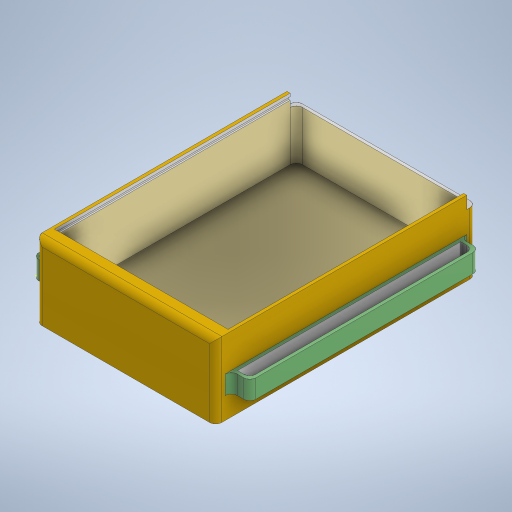
# Autodesk Inventor part: top
Saved by Autodesk Inventor 2023 (Build 270158000, 158)
## iProperties
Created: 2023-01-13
Part Number: top
Material: Generic
Document SubType Name: Modeling
Designer: zhanj390
Density: 1 g/cm^3
Appearance: Default
Author: zhanj390
Autodesk Inventor part; units mm, degrees
sketch "Sketch2" plane through (0, 0, 0) normal (0, 1, 0) x (-1, 0, 0)
  line L0 (0, 0) -> (-58, 0)
  line L1 (-58, 0) -> (-58, -84)
  line L2 (-58, -84) -> (0, -84)
  line L3 (0, -84) -> (0, 0)
  dimension "d0" = 58
  dimension "d1" = 84
  constraints: 8 end point, 2 parallel, 1 horizontal, 1 perpendicular
  measures "d0" distance of L1.end L2.end
  measures "d1" distance of L0.end L1.end
extrude "Extrusion1" add sketch "Sketch2" along normal blind 20
sketch "Sketch3" plane through (0, 20, 0) normal (0, 1, 0) x (1, 0, 0)
  line L0 (1, 1) -> (57, 1)
  line L1 (57, 1) -> (57, 83)
  line L2 (57, 83) -> (1, 83)
  line L3 (1, 83) -> (1, 1)
  line L4 (0, 84) -> (0, 0) projected
  line L5 (0, 0) -> (58, 0) projected
  line L6 (58, 84) -> (0, 84) projected
  line L7 (58, 0) -> (58, 84) projected
  dimension "d4" = 1
  dimension "d5" = 1
  dimension "d6" = 1
  dimension "d7" = 1
  constraints: 8 end point, 2 parallel, 1 horizontal, 1 perpendicular
  measures "d4" distance between parallel lines of L4 L3
  measures "d5" distance between parallel lines of L5 L0
  measures "d6" distance between parallel lines of L6 L2
  measures "d7" distance between parallel lines of L7 L1
extrude "Extrusion2" cut sketch "Sketch3" against normal blind 16 contours L3 L2 L1 L0
fillet "Fillet1" radius 2 4 edges at (0, 10, 0) (58, 10, 0) (58, 10, -84) (0, 10, -84)
ref_plane "Work Plane1" through (28, 20, -83) normal (-1, 0, 0) x (0, 0, 1)
sketch "Sketch17" plane through (58, 0, -2) normal (1, 0, 0) x (0, 0, -1)
  line L0 (3, 13) -> (77, 13)
  line L1 (77, 13) -> (77, 7)
  line L2 (77, 7) -> (3, 7)
  line L3 (3, 7) -> (3, 13)
  line L4 (0, 20) -> (80, 20) projected
  line L5 (0, 0) -> (80, 0) projected
  line L6 (80, 20) -> (80, 0) projected
  line L7 (0, 0) -> (0, 20) projected
  point P0 (-2, 0)
  point P1 (80, 10)
  point P2 (77, 10)
  point P3 (3, 10)
  dimension "d66" = 7
  dimension "d67" = 7
  dimension "d68" = 3
  dimension "d69" = 3
  constraints: 8 end point, 3 midpoint, 2 parallel, 1 horizontal, 1 perpendicular
  measures "d66" distance between parallel lines of L4 L0
  measures "d67" distance between parallel lines of L5 L2
  measures "d68" distance of point (80, 10) point (77, 10)
  measures "d69" distance from line of L7 point (3, 10)
extrude "Extrusion8" add sketch "Sketch17" along normal blind 6 contours L0 L1 L2 L3
sketch "Sketch18" plane through (58, 13, -5) normal (0, 1, 0) x (1, 0, 0)
  point P0 (-58, -5)
sketch "Sketch19" plane through (58, 13, -5) normal (0, 1, 0) x (1, 0, 0)
  line L0 (1, 73) -> (5, 73)
  line L1 (5, 73) -> (5, 1)
  line L2 (5, 1) -> (1, 1)
  line L3 (1, 1) -> (1, 73)
  line L4 (6, 74) -> (6, 0) projected
  line L5 (0, 0) -> (0, 74) projected
  line L6 (0, 0) -> (6, 0) projected
  line L7 (0, 74) -> (6, 74) projected
  point P0 (-58, -5)
  point P1 (3, 1)
  point P2 (3, 74)
  point P3 (3, 73)
  dimension "d72" = 1
  dimension "d73" = 1
  dimension "d74" = 1
  dimension "d75" = 1
  constraints: 8 end point, 3 midpoint, 2 parallel, 1 horizontal, 1 perpendicular
  measures "d72" distance between parallel lines of L4 L1
  measures "d73" distance between parallel lines of L5 L3
  measures "d74" distance from line of L6 point (3, 1)
  measures "d75" distance of point (3, 74) point (3, 73)
extrude "Extrusion9" cut sketch "Sketch19" against normal blind 6 contours L0 L1 L2 L3
fillet "Fillet4" radius 2 6 edges at (64, 10, -5) (64, 10, -79) (58, 10, -5) (58, 10, -79) (63, 10, -78) (63, 10, -6)
fillet "Fillet5" radius 2 4 edges at (1, 12, -83) (57, 12, -83) (57, 12, -1) (1, 12, -1)
ref_plane "Work Plane4" through (29, 0, -82) normal (-1, 0, 0) x (0, 0, 1)
mirror "Mirror2" about plane through (29, 0, -82) normal (-1, 0, 0) of "Extrusion8"
sketch "Sketch20" plane through (-6, 13, -79) normal (0, 1, 0) x (1, 0, 0)
  line L0 (5, -73) -> (1, -73)
  line L1 (1, -73) -> (1, -1)
  line L2 (1, -1) -> (5, -1)
  line L3 (5, -1) -> (5, -73)
  line L4 (6, -74) -> (0, -74) projected
  line L5 (0, 0) -> (0, -74) projected
  line L6 (6, 0) -> (6, -74) projected
  line L7 (6, 0) -> (0, 0) projected
  point P0 (6, -79)
  point P1 (3, -73)
  point P2 (3, -1)
  dimension "d80" = 1
  dimension "d81" = 1
  dimension "d82" = 1
  dimension "d83" = 1
  constraints: 8 end point, 2 midpoint, 2 parallel, 1 horizontal, 1 perpendicular
  measures "d80" distance from line of L4 point (3, -73)
  measures "d81" distance between parallel lines of L5 L1
  measures "d82" distance between parallel lines of L6 L3
  measures "d83" distance from line of L7 point (3, -1)
extrude "Extrusion10" cut sketch "Sketch20" against normal blind 6 contours L0 L1 L2 L3
fillet "Fillet6" radius 2 2 edges at (-6, 10, -5) (0, 10, -5)
fillet "Fillet7" radius 2 2 edges at (-6, 10, -79) (0, 10, -79)
ref_plane "Work Plane5" through (0, 20, 0) normal (0, 1, 0) x (1, 0, 0)
sketch "Sketch21" plane through (0, 20, 0) normal (0, 1, 0) x (1, 0, 0)
  line L0 (0, 82) -> (0, 2) projected
  line L1 (58, 0) -> (0, 0)
  line L2 (0, 0) -> (0, 5)
  line L3 (0, 5) -> (58, 5)
  line L4 (58, 5) -> (58, 0)
  line L5 (55, 1) -> (3, 1) projected
  line L6 (57, 81) -> (57, 3) projected
  line L7 (58, 5) -> (57, 5)
  line L8 (57, 5) -> (57, 81)
  line L9 (57, 81) -> (58, 81)
  line L10 (58, 81) -> (58, 5)
  line L11 (1, 3) -> (1, 81) projected
  line L12 (0, 5) -> (1, 5)
  line L13 (1, 5) -> (1, 81)
  line L14 (1, 81) -> (0, 81)
  line L15 (0, 81) -> (0, 5)
  point P0 (0, 0)
  point P1 (58, 2.5)
  point P2 (57, 5)
  point P3 (1, 5)
  point P4 (0, 81)
  dimension "d89" = 5
  dimension "d90" = 58
  dimension "d91" = 1
  constraints: 24 end point, 6 parallel, 3 horizontal, 3 perpendicular, 1 midpoint, 1 point on line
  measures "d89" distance between parallel lines of L1 L3
  measures "d90" distance from line of L0 point (58, 2.5)
  measures "d91" distance between parallel lines of L5 L1
extrude "Extrusion11" add sketch "Sketch21" along normal blind 4
sketch "Sketch22" plane through (57, 4, -81) normal (-1, 0, 0) x (0, 0, 1)
  line L0 (-3, 19) -> (76, 19)
  line L1 (76, 19) -> (76, 18)
  line L2 (76, 18) -> (-3, 18)
  line L3 (-3, 18) -> (-3, 19)
  line L4 (0, 16) -> (0, 20) projected
  line L5 (0, 20) -> (76, 20) projected
  line L6 (76, 16) -> (76, 20) projected
  point P0 (81, -4)
  point P1 (-3, 18.5)
  point P2 (76, 18.5)
  point P3 (-3, 16)
  dimension "d94" = 1
  dimension "d97" = 1
  dimension "d100" = 0
  dimension "d118" = 0
  constraints: 8 end point, 2 midpoint, 2 parallel, 1 horizontal, 1 perpendicular
  measures "d94" distance between parallel lines of L2 L0
  measures "d97" distance between parallel lines of L5 L0
  measures "d100" distance from line of L6 L0.end
  measures "d118" distance from line of point (-3, 16) L3
sketch "Sketch23" plane through (57, 20, -5) normal (0, 0, -1) x (-1, 0, 0)
  line L0 (0, 0) -> (56, 0) projected
  line L1 (54.7663, 0) -> (3.9216, 0)
  line L2 (0, 4) -> (56, 4) projected
  line L3 (0, 0) -> (0, 4) projected
  line L4 (0, 3) -> (56, 3)
  line L5 (56, 3) -> (56, 2)
  line L6 (56, 2) -> (0, 2)
  line L7 (0, 2) -> (0, 3)
  line L8 (56, 0) -> (56, 4) projected
  point P0 (57, -20)
  point P1 (0, 2.5)
  point P2 (0, 2)
  point P3 (0, 3)
  dimension "d102" = 1
  dimension "d104" = 0
  dimension "d105" = 1
  dimension "d106" = 0
  constraints: 10 end point, 2 parallel, 1 horizontal, 1 midpoint, 1 perpendicular, 1 point on line
  measures "d102" distance between parallel lines of L2 L4
  measures "d104" distance between parallel lines of L3 L7
  measures "d105" distance between parallel lines of L4 L6
  measures "d106" distance between parallel lines of L8 L5
extrude "Extrusion12" cut sketch "Sketch23" against normal blind 2 contours L3 L4 L5 L6
extrude "Extrusion13" cut sketch "Sketch22" against normal blind 0.5 contours L0 L4 L2 L3 | L0 L1 L2 L4
sketch "Sketch24" plane through (1, 4, -3) normal (1, 0, 0) x (0, 0, -1)
  line L0 (2, 19) -> (78, 19)
  line L1 (78, 19) -> (78, 18)
  line L2 (78, 18) -> (2, 18)
  line L3 (2, 18) -> (2, 19)
  line L4 (2, 19) -> (2, 20) projected
  line L5 (2, 20) -> (78, 20) projected
  line L6 (78, 16) -> (78, 20) projected
  point P0 (-3, -4)
  point P1 (2, 18.5)
  point P2 (78, 18.5)
  dimension "d111" = 1
  dimension "d112" = 0
  dimension "d113" = 1
  dimension "d114" = 0
  constraints: 8 end point, 2 midpoint, 2 parallel, 1 horizontal, 1 perpendicular
  measures "d111" distance between parallel lines of L2 L0
  measures "d112" distance from line of L4 point (2, 18.5)
  measures "d113" distance between parallel lines of L5 L0
  measures "d114" distance from line of L6 point (78, 18.5)
extrude "Extrusion14" cut sketch "Sketch24" against normal blind 0.5 contours L0 L1 L2 L3
fillet "Fillet8" radius 2 3 edges at (58, 22, 0) (0, 22, 0) (29, 24, 0)
body "Solid1"
